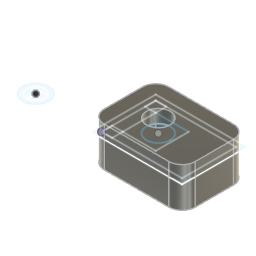
frame (Autodesk Fusion 360 design; units mm, degrees)
Autodesk Fusion 360 part; units mm, degrees
sketch "Sketch1" plane through (0, 0, 0) normal (0, 0, 1) x (1, 0, 0)
  line L0 (0, 0) -> (30.5, 0)
  line L1 (30.5, 0) -> (30.5, 20.5)
  line L2 (30.5, 20.5) -> (0, 20.5)
  line L3 (0, 20.5) -> (0, 0)
  line L4 (-2, -2) -> (32.5, -2)
  line L5 (32.5, -2) -> (32.5, 22.5)
  line L6 (32.5, 22.5) -> (-2, 22.5)
  line L7 (-2, 22.5) -> (-2, -2)
  line L8 (0, 20.5) -> (4, 20.5)
  line L9 (4, 20.5) -> (4, 16.5)
  line L10 (4, 16.5) -> (0, 16.5)
  line L11 (0, 16.5) -> (0, 20.5)
  line L12 (0, 0) -> (4, 0)
  line L13 (4, 0) -> (4, 4)
  line L14 (4, 4) -> (0, 4)
  line L15 (0, 4) -> (0, 0)
  line L16 (4, 4) -> (16.5, 4)
  line L17 (16.5, 4) -> (16.5, 16.5)
  line L18 (16.5, 16.5) -> (4, 16.5)
  line L19 (4, 16.5) -> (4, 4)
  circle A0 centre (11.25, 10.25) radius 4.5
  dimension "d1" = 30.5
  dimension "d2" = 20.5
  dimension "d3" = 2
  dimension "d4" = 4
  dimension "d5" = 4
  dimension "d6" = 4
  dimension "d7" = 4
  dimension "d8" = 12.5
  dimension "d9" = 9
  constraint horizontal L0
  constraint vertical L1
  constraint horizontal L2
  constraint vertical L3
  constraint coincident L0.start L3.end
  constraint horizontal L8
  constraint vertical L9
  constraint horizontal L10
  constraint vertical L11
  constraint horizontal L12
  constraint vertical L13
  constraint horizontal L14
  constraint vertical L15
  constraint horizontal L16
  constraint vertical L17
  constraint horizontal L18
  constraint vertical L19
  measures "d1" distance of L0.start L0.end
  measures "d2" distance of L0.start L2.end
  measures "d4" distance of L2.end L8.end
  measures "d5" distance of L2.end L10.end
  measures "d6" distance of L0.start L12.end
  measures "d7" distance of L0.start L14.end
  measures "d8" distance of L13.end L16.end
  measures "d9" diameter of A0
extrude "Extrude1" add sketch "Sketch1" along normal blind 2 contours L0 L3 L12 L13 L14 L15 | L0 L1 L2 L9 L13 L16 L17 L18 | L3 L10 L14 L19 | L16 L17 L18 L19 | L2 L3 L8 L9 L10 L11 | L4 L5 L6 L7
extrude "Extrude2" add sketch "Sketch1" against normal blind 10 contours L4 L5 L6 L7
fillet "Fillet1" radius 5 4 edges at (32.5, 22.5, -4) (32.5, -2, -4) (-2, -2, -4) (-2, 22.5, -4)
sketch "Sketch2" plane through (0, 0, 0) normal (0, 0, 1) x (1, 0, 0)
  circle A0 centre (-25, 0) radius 5
sketch "Sketch3" plane through (0, 0, 0) normal (0, 0, -1) x (1, 0, 0)
  circle A0 centre (-25, 0) radius 5
  circle A1 centre (-25, 0) radius 3.25
  line L0 (-25, 0) -> (-25, 3.25)
  line L1 (-25, 3.25) -> (-25, -1.75)
  line L2 (-25, -1.75) -> (-27.7386, -1.75)
  line L3 (-25, -1.75) -> (-22.2614, -1.75)
  dimension "d18" = 6.5
  dimension "d19" = 5
  constraint concentric A0 A1
  constraint coincident A0.centre A1.centre
  constraint coincident A1 L0.end
  constraint vertical L0
  constraint parallel L0 L1
  constraint coincident A1 L2.end
  constraint perpendicular L1 L2
  constraint coincident A1 L3.end
  constraint perpendicular L1 L3
  measures "d18" diameter of A1
  measures "d19" distance of L0.end L1.end
extrude "Extrude6" add 1 faces at (26.9167, 10.25, 2) along direction (0, 0, 1) blind 3
sketch "Sketch4" plane through (0, 0, 5) normal (0, 0, 1) x (-1, 0, 0)
  arc A0 (-3, -22.5) -> (2, -17.5) centre (-3, -17.5) ccw
  line L0 (2, -17.5) -> (2, -3)
  arc A1 (2, -3) -> (-3, 2) centre (-3, -3) ccw
  line L1 (-3, 2) -> (-27.5, 2)
  arc A2 (-27.5, 2) -> (-32.5, -3) centre (-27.5, -3) ccw
  line L2 (-32.5, -3) -> (-32.5, -17.5)
  arc A3 (-32.5, -17.5) -> (-27.5, -22.5) centre (-27.5, -17.5) ccw
  line L3 (-27.5, -22.5) -> (-3, -22.5)
  circle A4 centre (-11.25, -10.25) radius 4.5
sketch "Sketch5" plane through (0, 0, 5) normal (0, 0, 1) x (-1, 0, 0)
  circle A0 centre (8, 0) radius 5
sketch "Sketch6" plane through (0, -2, 0) normal (0, -1, 0) x (1, 0, 0)
  line L0 (3, 5) -> (3, -10)
  line L1 (3, -10) -> (27.5, -10)
  line L2 (27.5, -10) -> (27.5, 5)
  line L3 (27.5, 5) -> (3, 5)
sketch "Sketch7" plane through (0, 0, 5) normal (0, 0, 1) x (-1, 0, 0)
  arc A0 (-3, -22.5) -> (2, -17.5) centre (-3, -17.5) ccw
  line L0 (2, -17.5) -> (2, -3)
  arc A1 (2, -3) -> (-3, 2) centre (-3, -3) ccw
  line L1 (-3, 2) -> (-27.5, 2)
  arc A2 (-27.5, 2) -> (-32.5, -3) centre (-27.5, -3) ccw
  line L2 (-32.5, -3) -> (-32.5, -17.5)
  arc A3 (-32.5, -17.5) -> (-27.5, -22.5) centre (-27.5, -17.5) ccw
  line L3 (-27.5, -22.5) -> (-3, -22.5)
  circle A4 centre (-11.25, -10.25) radius 4.5
